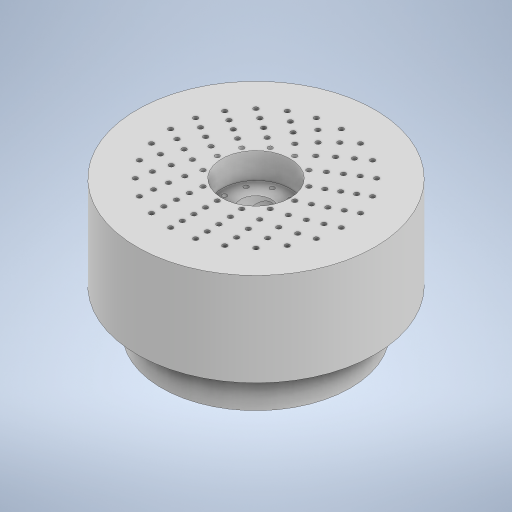
# Autodesk Inventor part: flyport_bottle_II
Saved by Autodesk Inventor 2023.1 (Build 271208000, 208)
## iProperties
Created: 2023-05-02
Part Number: flyport_bottle_II
Material: Generic
Document SubType Name: Modeling
Designer: dinesh
Density: 1 g/cm^3
Appearance: Default
Author: dinesh
Autodesk Inventor part; units mm, degrees
ref_plane "YZ Plane" through (0, 0, 0) normal (1, 0, 0) x (0, 1, 0)
ref_plane "XZ Plane" through (0, 0, 0) normal (0, 1, 0) x (-1, 0, 0)
ref_plane "XY Plane" through (0, 0, 0) normal (0, 0, 1) x (1, 0, 0)
sketch "Sketch1" plane through (0, 0, 0) normal (0, 0, 1) x (1, 0, 0)
  line L0 (3, 12) -> (23, 12)
  line L1 (23, 12) -> (23, 0)
  line L2 (3, 2) -> (3, 12)
  line L3 (0, 19.5472) -> (0, -22.4151)
  line L4 (23, 0) -> (22, 0) construction
  line L5 (22, 0) -> (22, -6)
  line L6 (22, -6) -> (23, -6)
  line L7 (23, -6) -> (23, 0)
  line L8 (20.4, 0) -> (17.25, 0) construction
  line L9 (17.25, 0) -> (17.25, -5) construction
  line L10 (17.25, -5) -> (20.4, -5) construction
  line L11 (20.4, -5) -> (20.4, 0)
  arc A0 (3, 2) -> (4.6637, 0.0285) centre (5, 2) ccw
  line L12 (22, 0) -> (20.4, 0)
  line L13 (17.25, 0) -> (5, 0)
  line L14 (-20.0393, 0) -> (22, 0) construction
  line L15 (23, 0) -> (24.5476, 0) construction
  line L16 (18.25, 0) -> (18.25, -5) construction
  line L17 (20.4, -5) -> (18.25, -5)
  line L18 (18.25, -5) -> (18.25, -14)
  line L19 (18.25, -14) -> (18.15, -14)
  line L20 (18.15, -14) -> (17.25, -5) construction
  line L21 (18.25, -8) -> (17.55, -8) construction
  line L22 (5.4025, -0.2566) -> (16.7316, -7.4783)
  line L23 (17.6466, -8.9658) -> (18.15, -14)
  arc A1 (17.6466, -8.9658) -> (16.7316, -7.4783) centre (15.6565, -9.1648) ccw
  arc A2 (5.4025, -0.2566) -> (4.6637, 0.0285) centre (4.3274, -1.943) ccw
  point P0 (0, 0)
  point P1 (17.25, 0)
  point P2 (17.25, -5)
  point P3 (5, 0)
  point P4 (17.9, -8)
  dimension "d0" = 6
  dimension "d2" = 1
  dimension "d5" = 5
  dimension "d6" = 1.6
  dimension "d7" = 44
  dimension "d11" = 2
  dimension "d12" = 12
  dimension "d14" = 6
  dimension "d23" = 36.5
  dimension "d24" = 1
  dimension "d25" = 0.1
  dimension "d26" = 9
  dimension "d37" = 3
  dimension "d38" = 2
  dimension "d39" = 2
  constraints: 48 end point, 14 point on line, 9 point on circle, 7 horizontal, 7 parallel, 6 collinear, 6 tangent, 5 perpendicular, 3 centre point, 3 vertical, 1 equal radius, 1 midpoint, 9 other
  measures "d0" diameter of L2 L3
  measures "d2" distance between parallel lines of L5 L7
  measures "d5" distance between parallel lines of L10 L8
  measures "d6" distance between parallel lines of L5 L11
  measures "d7" diameter of L5 L3
  measures "d11" radius of A0
  measures "d12" distance between parallel lines of L13 L0
  measures "d14" distance between parallel lines of L6 L4
  measures "d23" diameter of L16 L3
  measures "d25" distance of L18.end L19.end
  measures "d26" distance between parallel lines of L19 L10
  measures "d37" distance from line of point (17.9, -8) L10
  measures "d38" radius of A1
  measures "d39" radius of A2
revolve "Revolution1" add sketch "Sketch1" angle 360 about axis through (0, 19.5472, 0) along (0, -1, 0)
sketch "Sketch2" plane through (0, 0, 0) normal (0, 0, 1) x (1, 0, 0)
  line L0 (-3, 12) -> (3, 12) projected
  line L1 (0, 12) -> (0, 0) construction
  line L2 (-3, 2) -> (3, 2) construction
  circle A0 centre (0, 3.5) radius 3
  line L3 (-20.4, 0) -> (20.4, 0) projected
  point P0 (2.5981, 2)
  point P1 (-2.5981, 2)
  dimension "d16" = 6
  dimension "d40" = 3.5
  constraints: 2 end point, 1 centre point, 1 midpoint, 1 perpendicular, 1 point on line
  measures "d16" diameter of A0
  measures "d40" distance from line of L3 A0.centre
extrude "Extrusion1" cut sketch "Sketch2" along normal blind 3 and the other way blind 33
sketch "Sketch3" plane through (0, 12, 0) normal (0, 1, 0) x (1, 0, 0)
  circle A0 centre (0, 0) radius 6.6
  circle A1 centre (0, 0) radius 3 construction
  dimension "d27" = 13.2
  constraints: 1 centre point, 1 coincident, 1 concentric
  measures "d27" diameter of A0
extrude "Extrusion2" cut sketch "Sketch3" against normal blind 5
sketch "Sketch4" plane through (0, 12, 0) normal (0, 1, 0) x (1, 0, 0)
  circle A0 centre (0, 0) radius 3 projected
  circle A1 centre (0, 0) radius 23 projected
  line L0 (0, -23) -> (0, 23) construction
  line L1 (-23, 0) -> (23, 0) construction
  circle A2 centre (0, -5.25) radius 0.45
  circle A3 centre (0, -7.5) radius 0.45
  circle A4 centre (0, -14.25) radius 0.45
  circle A5 centre (0, -12) radius 0.45
  circle A6 centre (0, -9.75) radius 0.45
  circle A7 centre (0, -16.5) radius 0.45
  circle A8 centre (3.3746, -4.0217) radius 0.45
  circle A9 centre (5.1702, -0.9117) radius 0.45
  circle A10 centre (4.5466, 2.625) radius 0.45
  circle A11 centre (1.7956, 4.9334) radius 0.45
  circle A12 centre (-1.7956, 4.9334) radius 0.45
  circle A13 centre (3.75, -6.4952) radius 0.45
  circle A14 centre (6.4952, -3.75) radius 0.45
  circle A15 centre (7.5, 0) radius 0.45
  circle A16 centre (6.4952, 3.75) radius 0.45
  circle A17 centre (3.75, 6.4952) radius 0.45
  circle A18 centre (0, 7.5) radius 0.45
  circle A19 centre (-3.75, 6.4952) radius 0.45
  circle A20 centre (-6.4952, 3.75) radius 0.45
  circle A21 centre (3.9657, -8.9071) radius 0.45
  circle A22 centre (7.2457, -6.524) radius 0.45
  circle A23 centre (9.2728, -3.0129) radius 0.45
  circle A24 centre (9.6966, 1.0192) radius 0.45
  circle A25 centre (8.4437, 4.875) radius 0.45
  circle A26 centre (5.7309, 7.8879) radius 0.45
  circle A27 centre (2.0271, 9.5369) radius 0.45
  circle A28 centre (-2.0271, 9.5369) radius 0.45
  circle A29 centre (-5.7309, 7.8879) radius 0.45
  circle A30 centre (-8.4437, 4.875) radius 0.45
  circle A31 centre (-9.6966, 1.0192) radius 0.45
  circle A32 centre (4.1042, -11.2763) radius 0.45
  circle A33 centre (7.7135, -9.1925) radius 0.45
  circle A34 centre (10.3923, -6) radius 0.45
  circle A35 centre (11.8177, -2.0838) radius 0.45
  circle A36 centre (11.8177, 2.0838) radius 0.45
  circle A37 centre (10.3923, 6) radius 0.45
  circle A38 centre (7.7135, 9.1925) radius 0.45
  circle A39 centre (4.1042, 11.2763) radius 0.45
  circle A40 centre (0, 12) radius 0.45
  circle A41 centre (-4.1042, 11.2763) radius 0.45
  circle A42 centre (-7.7135, 9.1925) radius 0.45
  circle A43 centre (-10.3923, 6) radius 0.45
  circle A44 centre (-11.8177, 2.0838) radius 0.45
  circle A45 centre (-11.8177, -2.0838) radius 0.45
  circle A46 centre (4.2003, -13.6169) radius 0.45
  circle A47 centre (8.0273, -11.7739) radius 0.45
  circle A48 centre (11.1411, -8.8847) radius 0.45
  circle A49 centre (13.265, -5.2061) radius 0.45
  circle A50 centre (14.2102, -1.0649) radius 0.45
  circle A51 centre (13.8927, 3.1709) radius 0.45
  circle A52 centre (12.3409, 7.125) radius 0.45
  circle A53 centre (9.6925, 10.446) radius 0.45
  circle A54 centre (6.1828, 12.8388) radius 0.45
  circle A55 centre (2.1239, 14.0908) radius 0.45
  circle A56 centre (-2.1239, 14.0908) radius 0.45
  circle A57 centre (-6.1828, 12.8388) radius 0.45
  circle A58 centre (-9.6925, 10.446) radius 0.45
  circle A59 centre (-12.3409, 7.125) radius 0.45
  circle A60 centre (-13.8927, 3.1709) radius 0.45
  circle A61 centre (-14.2102, -1.0649) radius 0.45
  circle A62 centre (-13.265, -5.2061) radius 0.45
  circle A63 centre (4.2705, -15.9378) radius 0.45
  circle A64 centre (8.25, -14.2894) radius 0.45
  circle A65 centre (11.6673, -11.6673) radius 0.45
  circle A66 centre (14.2894, -8.25) radius 0.45
  circle A67 centre (15.9378, -4.2705) radius 0.45
  circle A68 centre (16.5, 0) radius 0.45
  circle A69 centre (15.9378, 4.2705) radius 0.45
  circle A70 centre (14.2894, 8.25) radius 0.45
  circle A71 centre (11.6673, 11.6673) radius 0.45
  circle A72 centre (8.25, 14.2894) radius 0.45
  circle A73 centre (4.2705, 15.9378) radius 0.45
  circle A74 centre (0, 16.5) radius 0.45
  circle A75 centre (-4.2705, 15.9378) radius 0.45
  circle A76 centre (-8.25, 14.2894) radius 0.45
  circle A77 centre (-11.6673, 11.6673) radius 0.45
  circle A78 centre (-14.2894, 8.25) radius 0.45
  circle A79 centre (-15.9378, 4.2705) radius 0.45
  circle A80 centre (-16.5, 0) radius 0.45
  circle A81 centre (-15.9378, -4.2705) radius 0.45
  circle A82 centre (-14.2894, -8.25) radius 0.45
  circle A83 centre (-4.5466, 2.625) radius 0.45
  circle A84 centre (-5.1702, -0.9117) radius 0.45
  circle A85 centre (-3.3746, -4.0217) radius 0.45
  circle A86 centre (-7.5, 0) radius 0.45
  circle A87 centre (-6.4952, -3.75) radius 0.45
  circle A88 centre (-3.75, -6.4952) radius 0.45
  circle A89 centre (-9.2728, -3.0129) radius 0.45
  circle A90 centre (-7.2457, -6.524) radius 0.45
  circle A91 centre (-3.9657, -8.9071) radius 0.45
  circle A92 centre (-10.3923, -6) radius 0.45
  circle A93 centre (-7.7135, -9.1925) radius 0.45
  circle A94 centre (-4.1042, -11.2763) radius 0.45
  circle A95 centre (-11.1411, -8.8847) radius 0.45
  circle A96 centre (-8.0273, -11.7739) radius 0.45
  circle A97 centre (-4.2003, -13.6169) radius 0.45
  circle A98 centre (-11.6673, -11.6673) radius 0.45
  circle A99 centre (-8.25, -14.2894) radius 0.45
  circle A100 centre (-4.2705, -15.9378) radius 0.45
  dimension "d41" = 0.9
  dimension "d42" = 0.9
  dimension "d43" = 0.9
  dimension "d44" = 0.9
  dimension "d45" = 0.9
  dimension "d47" = 5.25
  dimension "d48" = 2.25
  dimension "d49" = 2.25
  dimension "d50" = 2.25
  dimension "d51" = 2.25
  dimension "d52" = 0.9
  dimension "d53" = 2.25
  dimension "d56" = 360
  dimension "d60" = 360
  dimension "d64" = 360
  dimension "d68" = 360
  dimension "d72" = 360
  dimension "d76" = 360
  constraints: 99 centre point, 4 point on circle, 2 end point, 2 midpoint, 1 horizontal, 215 other
  measures "d41" diameter of A2
  measures "d42" diameter of A3
  measures "d43" diameter of A6
  measures "d44" diameter of A5
  measures "d45" diameter of A4
  measures "d47" distance of A2.centre A0.centre
  measures "d48" distance of A3.centre A2.centre
  measures "d49" distance of A6.centre A3.centre
  measures "d50" distance of A6.centre A5.centre
  measures "d51" distance of A5.centre A4.centre
  measures "d52" diameter of A7
  measures "d53" distance of A4.centre A7.centre
extrude "Extrusion3" cut sketch "Sketch4" against normal blind 18 contours A0 | A2 | A3 | A4 | A5 | A6 | A7 | A8 | A9 | A10 | A11 | A12 | A13 | A14 | A15 | A16 | A17 | A18 | A19 | A20 | A21 | A22 | A23 | A24 | A25 | A26 | A27 | A28 | A29 | A30 | A31 | A32 | A33 | A34 | A35 | A36 | A37 | A38 | A39 | A40 | A41 | A42 | A43 | A44 | A45 | A46 | A47 | A48 | A49 | A50 | A51 | A52 | A53 | A54 | A55 | A56 | A57 | A58 | A59 | A60 | A61 | A62 | A63 | A64 | A65 | A66 | A67 | A68 | A69 | A70 | A71 | A72 | A73 | A74 | A75 | A76 | A77 | A78 | A79 | A80 | A81 | A82 | A83 | A84 | A85 | A86 | A87 | A88 | A89 | A90 | A91 | A92 | A93 | A94 | A95 | A96 | A97 | A98 | A99 | A100
equation "\"d0\" = t_D"
equation "\"d2\" = w_th"
equation "\"d5\" = b_rim_h"
equation "\"d6\" = lv_th"
equation "\"d7\" = b_OD"
equation "\"d11\" = fillet_D"
equation "\"d12\" = top_th_f"
equation "\"d14\" = w_l"
equation "\"d23\" = b_ID"
equation "\"d24\" = w_th"
equation "\"d25\" = tol"
equation "\"d26\" = 1.5 * w_l"
equation "\"d37\" = 0.5 * w_l"
equation "\"d38\" = fillet_D"
equation "\"d39\" = fillet_D"
equation "\"d16\" = t_D"
equation "\"d40\" = 0.5 * w_th + 0.5 * t_D"
equation "\"d18\" = 0.5 * t_D"
equation "\"d19\" = 0.75 * b_OD"
equation "\"d27\" = cn_D"
equation "\"d30\" = cn_h"
equation "\"d41\" = h_D"
equation "\"d42\" = h_D"
equation "\"d43\" = h_D"
equation "\"d44\" = h_D"
equation "\"d45\" = h_D"
equation "\"d47\" = 0.5 * t_D + h_s"
equation "\"d48\" = h_s"
equation "\"d49\" = h_s"
equation "\"d50\" = h_s"
equation "\"d51\" = h_s"
equation "\"d52\" = h_D"
equation "\"d53\" = h_s"
equation "\"d78\" = top_th_f + w_l"
equation "\"tol\" = 0.1"
equation "\"fillet_D\" = 2"
equation "\"w_th\" = 1"
equation "\"w_l\" = 6"
equation "\"t_D\" = 6"
equation "\"t_D_f\" = t_D + w_th"
equation "\"top_th_f\" = t_D_f + cn_h"
equation "\"cn_h\" = 5"
equation "\"lv_th\" = 1.6"
equation "\"d3\" = w_l"
equation "\"d8\" = top_th_f"
equation "\"b_ID\" = 36.5"
equation "\"b_OD\" = 44"
equation "\"b_rim_h\" = 5"
equation "\"top_th\" = t_D + w_th"
equation "\"lv_OD\" = 26"
equation "\"sv_OD\" = 13"
equation "\"sv_th\" = 1.5"
equation "\"b_th\" = 1.5"
equation "\"h_s\" = 2.25"
equation "\"h_D\" = 0.9"
equation "\"v_h_D\" = 7.5"
equation "\"v_h_off\" = 0.5 * cn_D + 0.5 * v_h_D"
equation "\"cn_D\" = 13.2"
body "Solid1"
